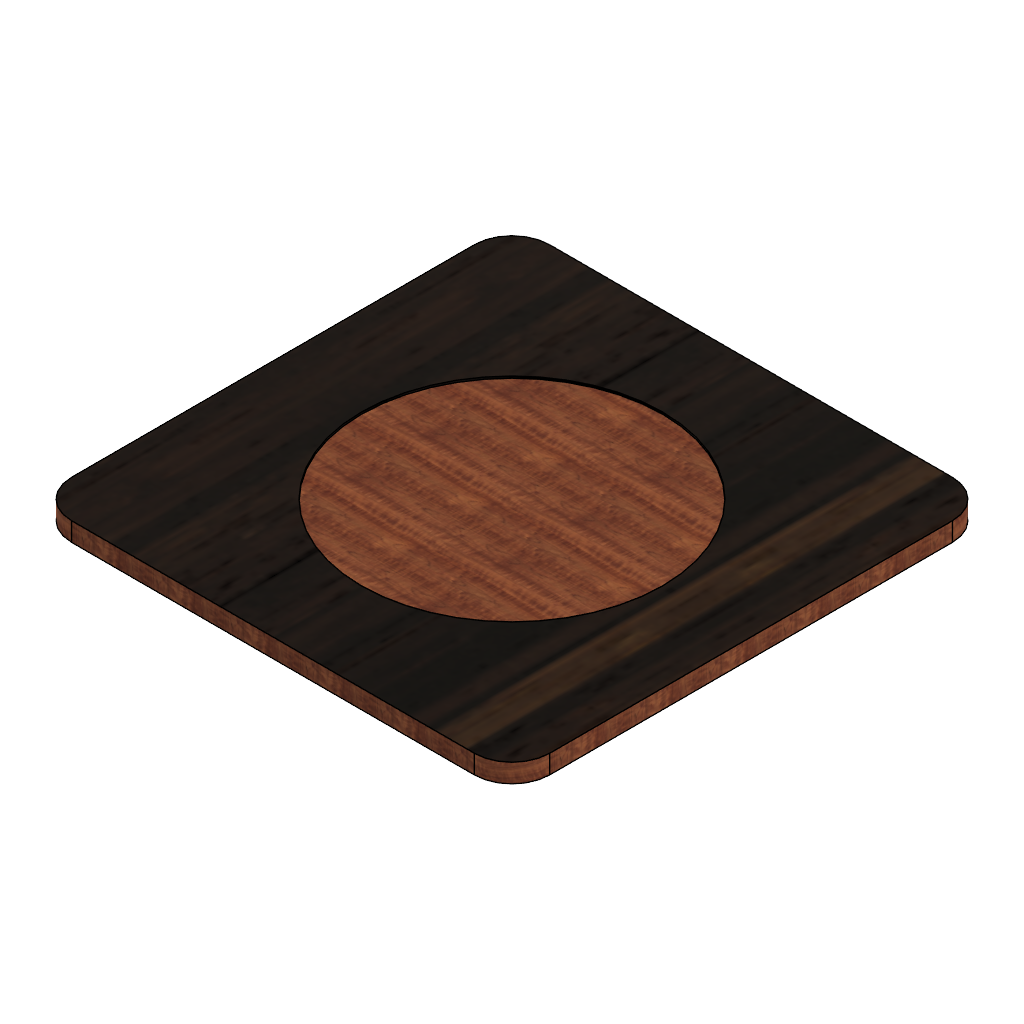
coaster (Autodesk Fusion 360 design; units mm, degrees)
Autodesk Fusion 360 part; units mm, degrees
sketch "Sketch1" plane through (0, 0, 0) normal (0, 0, 1) x (1, 0, 0)
  line L0 (63.5, -63.5) -> (-63.5, -63.5)
  line L1 (-63.5, -63.5) -> (-63.5, 63.5)
  line L2 (-63.5, 63.5) -> (63.5, 63.5)
  line L3 (63.5, 63.5) -> (63.5, -63.5)
  line L4 (63.5, -63.5) -> (-63.5, 63.5) construction
  line L5 (-63.5, -63.5) -> (63.5, 63.5) construction
  dimension "d1" = 127
  dimension "d2" = 127
  constraint horizontal L0
  constraint perpendicular L0 L1
  constraint parallel L0 L2
  constraint parallel L1 L3
  constraint coincident L4 origin
  constraint coincident L5 origin
  measures "d1" distance of L1.end L2.end
  measures "d2" distance of L0 L2
extrude "Extrude1" add sketch "Sketch1" along normal mid plane 5
chamfer "Chamfer1" distance 5 angle 45 4 edges at (-63.5, 63.5, 0) (-63.5, -63.5, 0) (63.5, 63.5, 0) (63.5, -63.5, 0) measured on face at (-21.1667, 63.5, -0.8333) measured on face at (-63.5, -21.1667, -0.8333) measured on face at (-21.1667, 63.5, -0.8333) measured on face at (-21.1667, -63.5, 0.8333)
fillet "Fillet1" radius 10 1 faces at (-61.8333, 60.1667, 0.8333)
fillet "Fillet2" radius 10 3 faces at (61.8333, -60.1667, -0.8333) (-60.1667, -61.8333, 0.8333) (61.8333, 60.1667, -0.8333)
sketch "Sketch2" plane through (0, 0, -2.5) normal (0, 0, -1) x (1, 0, 0)
  arc A0 (53.5, -63.5) -> (63.5, -53.5) centre (53.5, -53.5) ccw
  line L0 (63.5, -53.5) -> (63.5, 53.5)
  arc A1 (63.5, 53.5) -> (53.5, 63.5) centre (53.5, 53.5) ccw
  line L1 (53.5, 63.5) -> (-53.5, 63.5)
  arc A2 (-53.5, 63.5) -> (-63.5, 53.5) centre (-53.5, 53.5) ccw
  line L2 (-63.5, 53.5) -> (-63.5, -53.5)
  arc A3 (-63.5, -53.5) -> (-53.5, -63.5) centre (-53.5, -53.5) ccw
  line L3 (-53.5, -63.5) -> (53.5, -63.5)
  circle A4 centre (53.5, -53.5) radius 7.5
  circle A5 centre (-53.5, -53.5) radius 7.5
  circle A6 centre (53.5, 53.5) radius 7.5
  circle A7 centre (-53.5, 53.5) radius 7.5
  dimension "d11" = 15
  dimension "d12" = 15
  dimension "d13" = 15
  dimension "d14" = 15
  constraint concentric A0 A4
  constraint concentric A3 A5
  constraint concentric A1 A6
  constraint concentric A2 A7
  measures "d11" diameter of A4
  measures "d12" diameter of A6
  measures "d13" diameter of A5
  measures "d14" diameter of A7
extrude "Extrude2" add sketch "Sketch2" along normal blind 1 contours A4 | A5 | A6 | A7
cylinder "CylinderPrimitive2" cut diameter 80 height -0.5 placed x (1, 0, 0) y (0, 1, 0) z (0, 0, 1) at (0, 0, 2.5)
